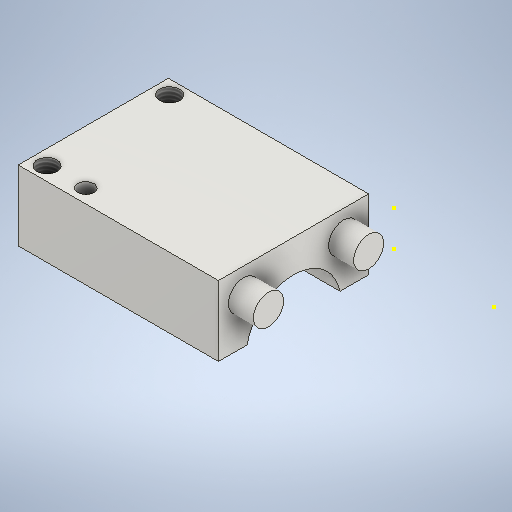
# Autodesk Inventor part: Rb oven housing top
Saved by Autodesk Inventor 2025.3 (Build 293356000, 356)
## iProperties
Created: 2025-04-11
Part Number: Rb oven housing top
Material: Generic
Document SubType Name: Modeling
Designer: Verðandi
Density: 1 g/cm^3
Appearance: Steel
Author: Verðandi
Autodesk Inventor part; units mm, degrees
ref_plane "YZ Plane" through (0, 0, 0) normal (1, 0, 0) x (0, 1, 0)
ref_plane "XZ Plane" through (0, 0, 0) normal (0, 1, 0) x (-1, 0, 0)
ref_plane "XY Plane" through (0, 0, 0) normal (0, 0, 1) x (1, 0, 0)
sketch "Sketch1" plane through (0, 0, 0) normal (0, 0, 1) x (1, 0, 0)
  line L0 (20, -7) -> (-20, -7)
  line L1 (-20, -7) -> (-20, 7)
  line L2 (-20, 7) -> (20, 7)
  line L3 (20, 7) -> (20, -7)
  line L4 (20, -7) -> (-20, 7) construction
  line L5 (-20, -7) -> (20, 7) construction
  point P0 (0, 0)
  dimension "d0" = 40
  dimension "d1" = 14
  constraints: 12 end point, 2 midpoint, 2 parallel, 1 horizontal, 1 perpendicular
  measures "d0" distance of L1.end L2.end
  measures "d1" distance of L0.end L1.end
extrude "Extrusion1" add sketch "Sketch1" along normal blind 30
sketch "Sketch2" plane through (20, -7, 0) normal (1, 0, 0) x (0, 0, -1)
  point P0 (0, 7)
sketch "Sketch3" plane through (20, -7, 0) normal (1, 0, 0) x (0, 0, -1)
  line L0 (0, 0) -> (-30, 0) projected
  line L1 (-15, 0) -> (-15, -2)
  arc A0 (-5.7129, 0) -> (-24.2871, 0) centre (-15, -2) ccw
  point P0 (0, 7)
  dimension "d4" = 2
  dimension "d5" = 19
  constraints: 2 end point, 2 point on circle, 2 point on line, 1 centre point, 1 coincident, 1 midpoint, 1 vertical
  measures "d4" distance of L1.start L1.end
  measures "d5" diameter of A0
extrude "Extrusion2" cut sketch "Sketch3" against normal blind 35
sketch "Sketch4" plane through (-20, 7, 0) normal (0, 1, 0) x (1, 0, 0)
  point P0 (20, 0)
sketch "Sketch5" plane through (-20, 7, 0) normal (0, 1, 0) x (1, 0, 0)
  line L0 (40, 0) -> (0, 0) projected
  line L1 (40, -30) -> (0, -30) projected
  line L2 (0, -30) -> (0, -27.25)
  line L3 (0, 0) -> (0, -30) projected
  line L4 (0, -27.25) -> (2.75, -27.25)
  circle A0 centre (2.75, -27.25) radius 2
  line L5 (0, 0) -> (0, -2.75)
  line L6 (0, -2.75) -> (2.75, -2.75)
  circle A1 centre (2.75, -2.75) radius 2
  line L7 (2.75, -27.25) -> (10.75, -27.25)
  circle A2 centre (10.75, -27.25) radius 1.5875
  point P0 (20, 0)
  dimension "d11" = 2.75
  dimension "d12" = 2.75
  dimension "d13" = 4
  dimension "d14" = 2.75
  dimension "d15" = 2.75
  dimension "d16" = 4
  dimension "d17" = 8
  dimension "d18" = 3.175
  constraints: 10 end point, 3 centre point, 3 coincident, 2 perpendicular, 2 point on line, 1 horizontal
  measures "d11" distance of L1.end L2.end
  measures "d12" distance of L2.end L4.end
  measures "d13" diameter of A0
  measures "d14" distance of L0.end L5.end
  measures "d15" distance of L5.end L6.end
  measures "d16" diameter of A1
  measures "d17" distance of L7.start L7.end
  measures "d18" diameter of A2
extrude "Extrusion3" cut sketch "Sketch5" against normal blind 100 contours A2
sketch "Sketch6" plane through (-20, 7, 0) normal (0, 1, 0) x (1, 0, 0)
  point P0 (20, 0)
sketch "Sketch7" plane through (20, -7, 0) normal (1, 0, 0) x (0, 0, -1)
  line L0 (0, 14) -> (-30, 14) projected
  line L1 (-30, 14) -> (-25, 14)
  line L2 (-25, 14) -> (-25, 9)
  line L3 (0, 14) -> (0, 0) projected
  line L4 (0, 14) -> (-5, 14)
  line L5 (-5, 14) -> (-5, 9)
  circle A0 centre (-25, 9) radius 3
  circle A1 centre (-5, 9) radius 3
  point P0 (0, 7)
  dimension "d21" = 5
  dimension "d22" = 5
  dimension "d23" = 5
  dimension "d24" = 5
  dimension "d25" = 6
  dimension "d26" = 6
  constraints: 8 end point, 2 centre point, 2 coincident, 2 point on line, 1 perpendicular, 1 vertical
  measures "d21" distance of L0.end L1.end
  measures "d22" distance of L1.end L2.end
  measures "d23" distance of L0.start L4.end
  measures "d24" distance of L4.end L5.end
  measures "d25" diameter of A0
  measures "d26" diameter of A1
extrude "Extrusion4" add sketch "Sketch7" along normal blind 5
move or copy body "Move Body1" bodies to move or copy 1 copy no translate (-20, 0, 0)
move or copy body "Move Body2" bodies to move or copy 1 copy no translate (-5, 0, 0)
sketch "Sketch8" plane through (0, 0, 0) normal (1, 0, 0) x (0, 1, 0)
  point P0 (0, 0)
sketch "Sketch9" plane through (-45, 7, 0) normal (0, 1, 0) x (1, 0, 0)
  line L0 (40, -30) -> (0, -30) projected
  line L1 (0, -30) -> (0, -27.25)
  line L2 (0, 0) -> (0, -30) projected
  line L3 (0, -27.25) -> (3, -27.25)
  circle A0 centre (3, -27.25) radius 2
  line L4 (0, 0) -> (0, -2.75)
  line L5 (0, -2.75) -> (3, -2.75)
  circle A1 centre (3, -2.75) radius 2
  point P0 (45, 0)
  dimension "d35" = 2.75
  dimension "d36" = 3
  dimension "d37" = 4
  dimension "d38" = 2.75
  dimension "d39" = 4
  dimension "d40" = 3
  constraints: 8 end point, 2 centre point, 2 coincident, 2 perpendicular, 2 point on line
  measures "d35" distance of L0.end L1.end
  measures "d36" distance of L1.end L3.end
  measures "d37" diameter of A0
  measures "d38" distance of L2.start L4.end
  measures "d39" diameter of A1
  measures "d40" distance of L4.end L5.end
extrude "Extrusion5" cut sketch "Sketch9" against normal blind 14
thread "Thread1" size "M4x0.7" class "6H" standard "ANSI Metric M Profile" full length
thread "Thread2" size "M4x0.7" class "6H" standard "ANSI Metric M Profile" full length
sketch "Sketch10" plane through (-5, -7, 0) normal (1, 0, 0) x (0, 0, -1)
  point P0 (0, 7)
body "Solid1"
